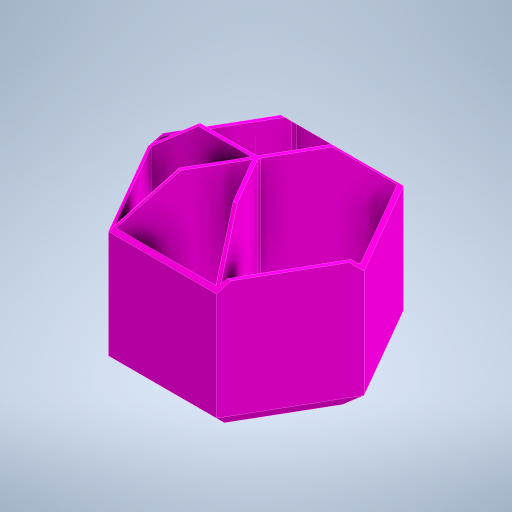
# Autodesk Inventor part: pen-pot
Saved by Autodesk Inventor 2023 (Build 270158030, 158C)
## iProperties
Created: 2024-08-23
Part Number: pen-pot
Material: Generic
Document SubType Name: Modeling
Designer: Imogen Heard
Density: 1 g/cm^3
Appearance: Magenta
Author: Imogen Heard
Autodesk Inventor part; units mm, degrees
ref_plane "YZ Plane" through (0, 0, 0) normal (1, 0, 0) x (0, 1, 0)
ref_plane "XZ Plane" through (0, 0, 0) normal (0, 1, 0) x (-1, 0, 0)
ref_plane "XY Plane" through (0, 0, 0) normal (0, 0, 1) x (1, 0, 0)
sketch "Sketch1" plane through (0, 0, 0) normal (0, 1, 0) x (-1, 0, 0)
  line L0 (-23.094, 40) -> (23.094, 40)
  line L1 (23.094, 40) -> (46.188, 0)
  line L2 (46.188, 0) -> (23.094, -40)
  line L3 (23.094, -40) -> (-23.094, -40)
  line L4 (-23.094, -40) -> (-46.188, 0)
  line L5 (-46.188, 0) -> (-23.094, 40)
  line L6 (0, 0) -> (62.8108, 0)
  line L7 (22.6615, -37.7492) -> (1.3, -0.75)
  line L8 (44.023, -0.75) -> (22.6615, -37.7492)
  line L9 (23.094, -40) -> (0, 0) construction
  line L10 (44.023, -0.75) -> (1.3, -0.75)
  line L11 (22.661, 37.75) -> (44.0225, 0.7508)
  line L12 (44.0225, 0.7508) -> (1.2995, 0.7508)
  line L13 (22.661, 37.75) -> (1.2995, 0.7508)
  line L14 (-21.362, 38.5) -> (21.361, 38.5)
  line L15 (21.361, 38.5) -> (-0.0005, 1.5008)
  line L16 (-21.362, 38.5) -> (-0.0005, 1.5008)
  line L17 (-44.023, 0.75) -> (-22.6615, 37.7492)
  line L18 (-22.6615, 37.7492) -> (-1.3, 0.75)
  line L19 (-44.023, 0.75) -> (-1.3, 0.75)
  line L20 (-22.661, -37.75) -> (-44.0225, -0.7508)
  line L21 (-44.0225, -0.7508) -> (-1.2995, -0.7508)
  line L22 (-22.661, -37.75) -> (-1.2995, -0.7508)
  line L23 (21.362, -38.5) -> (-21.361, -38.5)
  line L24 (-21.361, -38.5) -> (0.0005, -1.5008)
  line L25 (21.362, -38.5) -> (0.0005, -1.5008)
  point P0 (0, 0)
  point P1 (0, 0)
  dimension "d6" = 60
  dimension "d7" = 0.75
  dimension "d8" = 1.5
  dimension "d9" = 1.3
  dimension "d10" = 80
  dimension "d13" = 360
  constraints: 52 end point, 3 horizontal, 2 coincident, 1 horizontal alignment, 1 parallel, 50 other
  measures "d6" angle of L2 L7
  measures "d7" vertical distance of L1.end L8.start
  measures "d8" distance between parallel lines of L2 L8
  measures "d9" horizontal distance of point (0, 0) L7.end
  measures "d10" distance between parallel lines of L0 L3
extrude "Extrusion1" add sketch "Sketch1" along normal blind 70
sketch "Sketch2" plane through (0, 0, 0) normal (0, -1, 0) x (1, 0, 0)
  line L0 (23.094, 40) -> (46.188, 0) projected
  line L1 (-23.094, 40) -> (23.094, 40) projected
  line L2 (-46.188, 0) -> (-23.094, 40) projected
  line L3 (-23.094, -40) -> (-46.188, 0) projected
  line L4 (23.094, -40) -> (-23.094, -40) projected
  line L5 (46.188, 0) -> (23.094, -40) projected
  line L6 (-21.362, -38.5) -> (21.361, -38.5) projected
  line L7 (-0.0005, -1.5008) -> (-21.362, -38.5) projected
  line L8 (21.361, -38.5) -> (-0.0005, -1.5008) projected
  line L9 (22.661, -37.75) -> (44.0225, -0.7508) projected
  line L10 (1.2995, -0.7508) -> (22.661, -37.75) projected
  line L11 (44.0225, -0.7508) -> (1.2995, -0.7508) projected
  line L12 (44.023, 0.75) -> (22.6615, 37.7492) projected
  line L13 (1.3, 0.75) -> (44.023, 0.75) projected
  line L14 (22.6615, 37.7492) -> (1.3, 0.75) projected
  line L15 (21.362, 38.5) -> (-21.361, 38.5) projected
  line L16 (0.0005, 1.5008) -> (21.362, 38.5) projected
  line L17 (-21.361, 38.5) -> (0.0005, 1.5008) projected
  line L18 (-22.661, 37.75) -> (-44.0225, 0.7508) projected
  line L19 (-1.2995, 0.7508) -> (-22.661, 37.75) projected
  line L20 (-44.0225, 0.7508) -> (-1.2995, 0.7508) projected
  line L21 (-44.023, -0.75) -> (-22.6615, -37.7492) projected
  line L22 (-1.3, -0.75) -> (-44.023, -0.75) projected
  line L23 (-22.6615, -37.7492) -> (-1.3, -0.75) projected
  point P0 (0, 0)
extrude "Extrusion2" add sketch "Sketch2" along normal blind 3 contours L0 L5 L4 L3 L2 L1 | L7 L8 L6 | L10 L11 L9 | L13 L14 L12 | L16 L17 L15 | L19 L20 L18 | L22 L23 L21
sketch "Sketch4" plane through (0, 70, 0) normal (0, 1, 0) x (1, 0, 0)
  line L0 (23.094, -40) -> (46.188, 0) projected
  line L1 (46.188, 0) -> (23.094, 40) projected
  line L2 (23.094, 40) -> (-23.094, 40) projected
  line L3 (-23.094, 40) -> (-46.188, 0) projected
  line L4 (-46.188, 0) -> (-23.094, -40) projected
  line L5 (-23.094, -40) -> (23.094, -40) projected
  line L6 (-21.362, 38.5) -> (21.361, 38.5) projected
  line L7 (21.361, 38.5) -> (-0.0005, 1.5008) projected
  line L8 (-0.0005, 1.5008) -> (-21.362, 38.5) projected
  line L9 (22.661, 37.75) -> (44.0225, 0.7508) projected
  line L10 (44.0225, 0.7508) -> (1.2995, 0.7508) projected
  line L11 (1.2995, 0.7508) -> (22.661, 37.75) projected
  line L12 (44.023, -0.75) -> (22.6615, -37.7492) projected
  line L13 (22.6615, -37.7492) -> (1.3, -0.75) projected
  line L14 (1.3, -0.75) -> (44.023, -0.75) projected
  line L15 (21.362, -38.5) -> (-21.361, -38.5) projected
  line L16 (-21.361, -38.5) -> (0.0005, -1.5008) projected
  line L17 (0.0005, -1.5008) -> (21.362, -38.5) projected
  line L18 (-22.661, -37.75) -> (-44.0225, -0.7508) projected
  line L19 (-44.0225, -0.7508) -> (-1.2995, -0.7508) projected
  line L20 (-1.2995, -0.7508) -> (-22.661, -37.75) projected
  line L21 (-44.023, 0.75) -> (-22.6615, 37.7492) projected
  line L22 (-22.6615, 37.7492) -> (-1.3, 0.75) projected
  line L23 (-1.3, 0.75) -> (-44.023, 0.75) projected
  line L24 (-1.3, 0.75) -> (-44.023, 0.75) projected
  line L25 (-1.3, 0.75) -> (-0.0005, 1.5008)
  line L26 (-44.023, 0.75) -> (-22.6615, 37.7492) projected
  line L27 (-21.362, 38.5) -> (21.361, 38.5) projected
  line L28 (-22.6615, 37.7492) -> (-21.362, 38.5)
  constraints: 4 end point
extrude "Extrusion3" cut sketch "Sketch4" against normal up to surface (70 mm away) contours L8 L25 L22 L28
pattern_circular "Circular Pattern1" count 2 over 240 about axis through (0, -10, 0) along (0, 1, 0) of "Extrusion3"
chamfer "Chamfer2" distance 7 angle 45 6 edges at (-0.0005, 0, -38.5) (33.3417, 0, -19.2504) (33.3422, 0, 19.2496) (0.0005, 0, 38.5) (-33.3417, 0, 19.2504) (-33.3422, 0, -19.2496)
chamfer "Chamfer1" distance 8 angle 45 6 edges at (34.641, -3, -20) (34.641, -3, 20) (0, -3, 40) (-34.641, -3, 20) (-34.641, -3, -20) (0, -3, -40)
chamfer "Chamfer3" distance 19 angle 45 2 edges at (34.641, 70, -20) (0, 70, -40)
chamfer "Chamfer4" distance 19 angle 45 2 edges at (0, 70, 40) (-34.641, 70, 20)
sketch "Sketch5" plane through (0, 70, 0) normal (0, 1, 0) x (1, 0, 0)
  line L0 (34.0637, -21) -> (32.3316, -21) projected
  line L1 (34.0637, -21) -> (35.2184, -19) projected
  line L2 (34.3523, -17.5) -> (35.2184, -19) projected
  line L3 (34.3523, -17.5) -> (32.3316, -21) projected
  line L4 (-34.3523, 17.5) -> (-35.2184, 19) projected
  line L5 (-34.3523, 17.5) -> (-32.3316, 21) projected
  line L6 (-34.0637, 21) -> (-32.3316, 21) projected
  line L7 (-34.0637, 21) -> (-35.2184, 19) projected
  line L8 (-23.094, 40) -> (-34.0637, 21) projected
  line L9 (-34.0637, 21) -> (-32.3316, 21) projected
  line L10 (-32.3316, 21) -> (-22.6615, 37.7492) projected
  line L11 (-22.6615, 37.7492) -> (-21.362, 38.5) projected
  line L12 (-21.362, 38.5) -> (21.361, 38.5) projected
  line L13 (21.361, 38.5) -> (11.2574, 21) projected
  line L14 (11.2574, 21) -> (12.1244, 21) projected
  line L15 (12.1244, 21) -> (23.094, 40) projected
  line L16 (23.094, 40) -> (-23.094, 40) projected
  line L17 (-35.2184, 19) -> (-46.188, 0) projected
  line L18 (-46.188, 0) -> (-23.094, -40) projected
  line L19 (-23.094, -40) -> (-12.1244, -21) projected
  line L20 (-12.1244, -21) -> (-12.5574, -20.25) projected
  line L21 (-12.5574, -20.25) -> (-22.661, -37.75) projected
  line L22 (-22.661, -37.75) -> (-44.0225, -0.7508) projected
  line L23 (-44.0225, -0.7508) -> (-23.8152, -0.7508) projected
  line L24 (-23.8152, -0.7508) -> (-24.6817, 0.75) projected
  line L25 (-24.6817, 0.75) -> (-44.023, 0.75) projected
  line L26 (-44.023, 0.75) -> (-34.3523, 17.5) projected
  line L27 (-34.3523, 17.5) -> (-35.2184, 19) projected
  line L28 (12.1244, 21) -> (23.094, 40) projected
  line L29 (12.1244, 21) -> (12.5574, 20.25) projected
  line L30 (12.5574, 20.25) -> (22.661, 37.75) projected
  line L31 (22.661, 37.75) -> (44.0225, 0.7508) projected
  line L32 (44.023, -0.75) -> (34.3523, -17.5) projected
  line L33 (34.3523, -17.5) -> (35.2184, -19) projected
  line L34 (35.2184, -19) -> (46.188, 0) projected
  line L35 (46.188, 0) -> (23.094, 40) projected
  line L36 (-23.094, -40) -> (-12.1244, -21) projected
  line L37 (-23.094, -40) -> (23.094, -40) projected
  line L38 (23.094, -40) -> (34.0637, -21) projected
  line L39 (34.0637, -21) -> (32.3316, -21) projected
  line L40 (32.3316, -21) -> (22.6615, -37.7492) projected
  line L41 (22.6615, -37.7492) -> (12.9913, -21) projected
  line L42 (12.9913, -21) -> (11.2583, -21) projected
  line L43 (11.2583, -21) -> (21.362, -38.5) projected
  line L44 (21.362, -38.5) -> (-21.361, -38.5) projected
  line L45 (-21.361, -38.5) -> (-11.2574, -21) projected
  line L46 (-11.2574, -21) -> (-12.1244, -21) projected
  line L47 (44.023, -0.75) -> (45.755, -0.75)
  line L48 (22.6615, -37.7492) -> (23.5275, -39.2492)
  line L49 (-22.6615, 37.7492) -> (-23.5275, 39.2492)
  line L50 (-44.023, 0.75) -> (-45.755, 0.75)
  line L51 (0.0005, -1.5008) -> (11.2583, -21) projected
  line L52 (44.0225, 0.7508) -> (44.023, -0.75) projected
  point P0 (0, 0)
  constraints: 8 end point, 4 point on line, 2 horizontal, 1 collinear, 1 parallel
extrude "Extrusion4" cut sketch "Sketch5" against normal blind 15 contours L38 L48 L40 L0 | L0 L3 L2 L1 | L2 L32 L47 L34 | L17 L4 L26 L50 | L49 L10 L6 L8 | L7 L6 L5 L4
sketch "Sketch6" plane through (0, 70, 0) normal (0, 1, 0) x (1, 0, 0)
  circle A0 centre (-14.6939, 17.2494) radius 16
  ellipse E0 centre (24.2145, -2.943) end of major axis (24.1547, -26.9429) minor radius 17.5
  point P0 (0, 0)
  dimension "d37" = 24
  dimension "d38" = 17.5
  dimension "d36" = 32
  constraints: 1 centre point, 2 other
  measures "d36" diameter of A0
